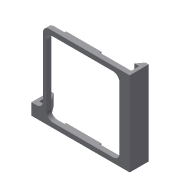
# Autodesk Inventor part: 30_Cube_Insert_Filter_Revolver_Filter_clamp_v3
Saved by Autodesk Inventor 2019.4 (Build 234330000, 330)
## iProperties
Created: 2021-09-14
Part Number: 30_Cube_Insert_Filter_Revolver_Filter_clamp_v3
Material: Generic
Document SubType Name: Modeling
Designer: diederichbenedict
Density: 1 g/cm^3
Appearance: Default
Mass: 0.70962 g
Surface Area: 14.1923 cm^2
Volume: 0.70962 cm^3
Author: diederichbenedict
Autodesk Inventor part; units mm, degrees
ref_plane "YZ Plane" through (0, 0, 0) normal (1, 0, 0) x (0, 1, 0)
ref_plane "XZ Plane" through (0, 0, 0) normal (0, 1, 0) x (-1, 0, 0)
ref_plane "XY Plane" through (0, 0, 0) normal (0, 0, 1) x (1, 0, 0)
sketch "Sketch1" plane through (0, 0, 0) normal (0, 1, 0) x (-1, 0, 0)
  line L0 (-2.8219, -9.5942) -> (-2.8219, -5.0355) construction
  line L1 (-28.25, -5.0355) -> (-2.8219, -5.0355) construction
  line L2 (-28.25, -5.0355) -> (-28.25, -24.4992) construction
  line L3 (-28.25, -24.4992) -> (-2.8219, -24.4992) construction
  line L4 (-2.8219, -24.4992) -> (-2.8219, -19.0192) construction
  ellipse E0 centre (-13.75, -14.3067) end of major axis (-0.95, -14.3067) minor radius 9.051 (-2.8219, -9.5942) -> (-2.8219, -19.0192) ccw construction
  line L5 (-26.25, -1.5) -> (-1.25, -1.5) construction
  line L6 (-1.25, -1.5) -> (-1.25, -0.5) construction
  line L7 (-26.25, -0.5) -> (-1.25, -0.5) construction
  line L8 (-26.25, -1.5) -> (-26.25, -0.5) construction
  line L9 (-29.47, 1.1) -> (1.53, 1.1)
  line L10 (1.53, 1.1) -> (1.53, -0.4)
  line L11 (1.53, -0.4) -> (-29.47, -0.4)
  line L12 (-29.47, -0.4) -> (-29.47, 1.1)
  line L13 (-29.47, -0.4) -> (-28.47, -0.4)
  line L14 (-28.47, -0.4) -> (-28.47, -4.9)
  line L15 (-28.47, -4.9) -> (-29.47, -4.9)
  line L16 (-29.47, -4.9) -> (-29.47, -0.4)
  line L17 (1.53, -0.4) -> (0.53, -0.4)
  line L18 (0.53, -0.4) -> (0.53, -4.9)
  line L19 (0.53, -4.9) -> (1.53, -4.9)
  line L20 (1.53, -4.9) -> (1.53, -0.4)
  line L21 (-28.47, -2.9) -> (-26.97, -2.9)
  line L22 (-26.97, -2.9) -> (-28.47, -4.9)
  line L23 (0.53, -2.9) -> (-0.97, -2.9)
  line L24 (-0.97, -2.9) -> (0.53, -4.9)
  point P0 (0, 0)
  dimension "d4" = 0.1
  dimension "d5" = 1.5
  dimension "d6" = 1
  dimension "d7" = 1
  dimension "d23" = 29
  dimension "d24" = 2
  dimension "d25" = 1.5
  dimension "d26" = 1.5
  dimension "d27" = 2
  dimension "d28" = 2.5
  constraints: 32 end point, 6 parallel, 6 point on line, 4 horizontal, 3 perpendicular, 1 other
  measures "d4" distance between parallel lines of L11 L7
  measures "d5" distance between parallel lines of L11 L9
  measures "d6" distance between parallel lines of L14 L12
  measures "d7" distance between parallel lines of L18 L20
  measures "d23" distance between parallel lines of L18 L14
  measures "d24" distance from line of L18.end L23
  measures "d25" distance of L23.start L23.end
  measures "d26" distance of L21.start L21.end
  measures "d27" distance from line of L22.end L21
  measures "d28" distance between parallel lines of L11 L23
extrude "Extrusion1" add sketch "Sketch1" along normal blind 15 and the other way blind 11.5
sketch "Sketch2" plane through (-1.53, 15, 1.1) normal (0, 0, 1) x (1, 0, 0)
  ellipse E0 centre (16.28, -15.0787) end of major axis (16.28, -13.4102) minor radius 1.1798 (15.3155, -14.1177) -> (17.2444, -14.1177) ccw projected
  arc A0 (15.1547, -13.58) -> (15.3155, -14.1177) centre (16.28, -13.5363) ccw projected
  ellipse E1 centre (16.28, -13.0787) end of major axis (16.28, -11.4102) minor radius 1.1798 (17.4052, -13.58) -> (15.1547, -13.58) ccw projected
  arc A1 (17.2444, -14.1177) -> (17.4052, -13.58) centre (16.28, -13.5363) ccw projected
  ellipse E2 centre (3.78, -31.5363) end of major axis (3.78, -30.2787) minor radius 0.8893 (4.6692, -31.5363) -> (3.78, -30.2787) ccw projected
  line L0 (4.6692, -31.5363) -> (27.5745, -31.5363) projected
  ellipse E3 centre (28.78, -31.5363) end of major axis (28.78, -29.8315) minor radius 1.2055 (28.78, -29.8315) -> (27.5745, -31.5363) ccw projected
  line L1 (28.78, -29.8315) -> (28.78, 4.4637) projected
  line L2 (28.78, 4.4637) -> (3.78, 4.4637) projected
  line L3 (3.78, 4.4637) -> (3.78, -30.2787) projected
  line L4 (31, -26.5) -> (31, 0) construction
  line L5 (0, 0) -> (31, 0) construction
  line L6 (0, 0) -> (0, -26.5) construction
  line L7 (31, -26.5) -> (0, -26.5) construction
  line L8 (4.78, -1.5) -> (27.78, -1.5)
  line L9 (27.78, -1.5) -> (27.78, -25)
  line L10 (27.78, -25) -> (4.78, -25)
  line L11 (4.78, -25) -> (4.78, -1.5)
  line L12 (4.78, -1.5) -> (27.78, -25) construction
  line L13 (27.78, -1.5) -> (4.78, -25) construction
  point P0 (16.28, -13.25)
  dimension "d19" = 1.5
  dimension "d20" = 1.5
  dimension "d21" = 1
  dimension "d22" = 1
  constraints: 12 end point, 2 midpoint, 2 parallel, 1 horizontal, 1 perpendicular, 4 other
  measures "d19" distance between parallel lines of L10 L7
  measures "d20" distance between parallel lines of L8 L5
  measures "d21" distance between parallel lines of L1 L9
  measures "d22" distance between parallel lines of L3 L11
extrude "Extrusion2" cut sketch "Sketch2" against normal blind 14 contours A0 E1 A1 E0 | L8 L9 L10 L11
fillet "Fillet1" radius 2 4 edges at (26.25, 13.5, 0.35) (26.25, -10, 0.35) (3.25, -10, 0.35) (3.25, 13.5, 0.35)
sketch "Sketch3" plane through (28.47, -11.5, -0.4) normal (0, 0, -1) x (-1, 0, 0)
  line L0 (25.22, 23) -> (25.22, 3.5) projected
  arc A0 (23.22, 1.5) -> (25.22, 3.5) centre (23.22, 3.5) ccw projected
  line L1 (23.22, 1.5) -> (4.22, 1.5) projected
  arc A1 (2.22, 3.5) -> (4.22, 1.5) centre (4.22, 3.5) ccw projected
  line L2 (2.22, 3.5) -> (2.22, 23) projected
  arc A2 (4.22, 25) -> (2.22, 23) centre (4.22, 23) ccw projected
  line L3 (4.22, 25) -> (23.22, 25) projected
  arc A3 (25.22, 23) -> (23.22, 25) centre (23.22, 23) ccw projected
  line L4 (0, 26.5) -> (0, 0) projected
  line L5 (29, 0) -> (0, 0) projected
  line L6 (29, 26.5) -> (29, 0) projected
  line L7 (0, 26.5) -> (29, 26.5) projected
  line L8 (30, 26.5) -> (-1, 26.5) projected
  line L9 (23.22, 25) -> (4.22, 25) projected
  line L10 (21.0097, 26.5) -> (9.9335, 26.5)
  line L11 (9.9335, 26.5) -> (9.9335, 25)
  line L12 (9.9335, 25) -> (21.0097, 25)
  line L13 (21.0097, 25) -> (21.0097, 26.5)
  line L14 (4.22, 1.5) -> (23.22, 1.5) projected
  line L15 (29, 0) -> (0, 0) projected
  line L16 (21.0097, 1.5) -> (9.9335, 1.5)
  line L17 (9.9335, 1.5) -> (9.9335, 0)
  line L18 (9.9335, 0) -> (21.0097, 0)
  line L19 (21.0097, 0) -> (21.0097, 1.5)
  point P0 (28.47, 11.5)
  constraints: 16 end point, 6 point on line, 4 parallel, 2 horizontal, 2 perpendicular
extrude "Extrusion3" add sketch "Sketch3" along normal blind 0.5 contours L3 L11 L7 L13 | L19 L5 L17 L1
sketch "Sketch4" plane through (-0.53, -11.5, -0.4) normal (0, 0, -1) x (-1, 0, 0)
  line L0 (-7.9903, 26.5) -> (-7.9903, 25) projected
  line L1 (-7.9903, 25) -> (-5.78, 25) projected
  arc A0 (-3.78, 23) -> (-5.78, 25) centre (-5.78, 23) ccw projected
  line L2 (-3.78, 23) -> (-3.78, 3.5) projected
  arc A1 (-5.78, 1.5) -> (-3.78, 3.5) centre (-5.78, 3.5) ccw projected
  line L3 (-5.78, 1.5) -> (-7.9903, 1.5) projected
  line L4 (-7.9903, 1.5) -> (-7.9903, 0) projected
  line L5 (0, 0) -> (-7.9903, 0) projected
  line L6 (0, 26.5) -> (0, 0) projected
  line L7 (-7.9903, 26.5) -> (0, 26.5) projected
  line L8 (-2.6734, 28.8214) -> (7.6365, 28.8214)
  line L9 (7.6365, 28.8214) -> (7.6365, 3.668)
  line L10 (7.6365, 3.668) -> (-2.6734, 3.668)
  line L11 (-2.6734, 3.668) -> (-2.6734, 28.8214)
  point P0 (-0.53, 11.5)
  constraints: 8 end point, 2 parallel, 1 horizontal, 1 perpendicular
extrude "Extrusion4" cut sketch "Sketch4" along normal through all both and the other way through all contours L11 L8 L9 L10 L6 L7 | L7 L6 L10 L11
fillet "Fillet2" radius 2 2 edges at (2.1434, -7.832, 0.35) (2.1434, 15, 0.35)
body "Solid1"
